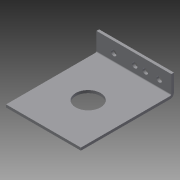
# Autodesk Inventor part: New Bracket for arm motor
Saved by Autodesk Inventor 2013 (Build 170138000, 138)
## iProperties
Created: 2013-01-31
Part Number: New Bracket for arm motor
Material: Generic
Document SubType Name: Sheet Metal
Designer: aslane
Density: 1 g/cm^3
Sheet Metal Rule: Default
Author: aslane
Autodesk Inventor part; units mm, degrees
ref_plane "YZ Plane" through (0, 0, 0) normal (1, 0, 0) x (0, 1, 0)
ref_plane "XZ Plane" through (0, 0, 0) normal (0, 1, 0) x (-1, 0, 0)
ref_plane "XY Plane" through (0, 0, 0) normal (0, 0, 1) x (1, 0, 0)
sketch "Sketch3" plane through (0, 0, 0) normal (0, 1, 0) x (-1, 0, 0)
  line L0 (0, 0) -> (90, 0)
  line L1 (90, 0) -> (90, 86.54)
  line L2 (90, 86.54) -> (0, 86.54)
  line L3 (0, 86.54) -> (0, 0)
  line L4 (0, 0) -> (0, -25.4)
  line L5 (0, -25.4) -> (90, -25.4)
  line L6 (90, -25.4) -> (90, 0)
  dimension "d13" = 90
  dimension "d14" = 86.54
  dimension "d15" = 25.4
  measures "d13" distance of L0.start L0.end
  measures "d14" distance of L0.end L1.end
  measures "d15" distance of L0.start L4.end
extrude "Plate3" add sketch "Sketch3" along normal blind 3.175
sketch "Sketch4" plane through (-90, 0, -22.225) normal (0, 0, -1) x (-1, 0, 0)
  line L0 (-90, 0) -> (0, 0)
  line L1 (0, 0) -> (0, 25.4)
  line L2 (0, 25.4) -> (-90, 25.4)
  line L3 (-90, 25.4) -> (-90, 0)
  constraints: 6 end point, 1 horizontal, 1 perpendicular, 1 vertical
edge flange "Flange2" height 25.4 angle 90 thickness 3.175 bend radius 1.27 thickness toward (0, 0, -1) relief tear relief width 3.175 relief depth 1.5875 edges at (-45, 3.175, -25.4) wall of the first edge with corners at (0, 0, -22.225) (-90, 0, -22.225) (-90, 25.4, -22.225) (0, 25.4, -22.225)
bend "Bend2"
corner "Corner2"
sketch "Sketch5" plane through (0, 3.175, 0) normal (0, 1, 0) x (1, 0, 0)
  line L0 (0, 20.955) -> (-90, 20.955) projected
  line L1 (-90, -86.54) -> (-90, 20.955) projected
  line L2 (0, -86.54) -> (-90, -86.54) projected
  line L3 (0, 20.955) -> (0, -86.54) projected
  line L4 (-45, 20.955) -> (-45, -86.54)
  line L5 (0, -32.7925) -> (-90, -32.7925)
  circle A0 centre (-45, -32.7925) radius 15
  point P0 (0, 0)
  dimension "d27" = 30
  constraints: 5 midpoint, 4 end point, 1 centre point
  measures "d27" diameter of A0
extrude "Cut1" cut sketch "Sketch5" against normal blind 3.175 contours A0 L5 L4 | L4 L5 A0 | A0 L4 L5 | L4 A0 L5
sketch "Sketch6" plane through (-90, 25.4, -22.225) normal (0, 0, 1) x (1, 0, 0)
  circle A0 centre (20.701, -12.7) radius 3.302 projected
  circle A1 centre (58.801, -12.7) radius 3.302 projected
  circle A2 centre (46.101, -12.7) radius 3.302 projected
  circle A3 centre (1.651, -12.7) radius 3.302 projected
  circle A4 centre (119.9021, -12.7) radius 3.302 projected
  circle A5 centre (75.4521, -12.7) radius 3.302 projected
  point P0 (90, -25.4)
extrude "Cut2" cut sketch "Sketch6" against normal blind 3.175 contours A0 | A1 | A2 | A5
equation "\"d28\" = Thickness"
equation "\"d30\" = Thickness"
equation "\"d17\" = BendReliefWidth"
equation "\"d18\" = BendReliefDepth"
equation "\"d19\" = MinimumRemnant"
equation "\"d20\" = BendRadius"
equation "\"d24\" = CornerReliefSize"
equation "\"d25\" = GapSize"
equation "\"d26\" = JacobiRadiusSize"
equation "\"BendRadius\" = Thickness"
equation "\"BendReliefWidth\" = Thickness"
equation "\"BendReliefDepth\" = 0.5 * Thickness"
equation "\"CornerReliefSize\" = 4 * Thickness"
equation "\"MinimumRemnant\" = 2 * Thickness"
equation "\"TransitionRadius\" = BendRadius"
equation "\"JacobiRadiusSize\" = BendRadius"
equation "\"GapSize\" = Thickness"
equation "\"d2\" = BendRadius"
equation "\"d16\" = BendRadius"
equation "\"Thickness\" = 3.175"
body "Solid2"
